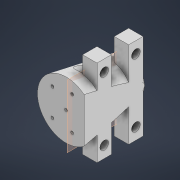
# Autodesk Inventor part: needle module it 5
Saved by Autodesk Inventor 2022 (Build 260153000, 153)
## iProperties
Created: 2023-02-14
Part Number: needle module it 5
Material: Generic
Document SubType Name: Modeling
Designer: Jakob Saugbjerg
Density: 1 g/cm^3
Appearance: Default
Author: Jakob Saugbjerg
Autodesk Inventor part; units mm, degrees
ref_plane "YZ Plane" through (0, 0, 0) normal (1, 0, 0) x (0, 1, 0)
sketch "Sketch1" plane through (0, 0, 0) normal (0, 0, 1) x (1, 0, 0)
  circle A0 centre (0, 0) radius 6.25
  dimension "d1" = 12.5
  constraints: 1 centre point, 1 coincident
  measures "d1" diameter of A0
extrude "Extrusion1" add sketch "Sketch1" along normal blind 21 draft 10
sketch "Sketch2" plane through (0, 0, 0) normal (0, 0, -1) x (-1, 0, 0)
  circle A0 centre (0, 0) radius 6.25 projected
  line L0 (-6.25, 0) -> (-13, 0)
  line L1 (-13, 0) -> (-13, -18)
  line L2 (-13, -18) -> (-6.25, -18)
  line L3 (-6.25, -18) -> (-6.25, 0)
  line L4 (-6.25, 0) -> (-13, 0)
  line L5 (-13, 0) -> (-13, 12)
  line L6 (-13, 12) -> (-6.25, 12)
  line L7 (-6.25, 12) -> (-6.25, 0)
  constraints: 16 end point, 4 parallel, 2 horizontal, 2 perpendicular, 1 horizontal alignment, 1 other
extrude "Extrusion2" cut sketch "Sketch2" against normal blind 21 contours L3 L2 L1 L0 | L0 L5 L6 L7
sketch "Sketch3" plane through (0, 0, 0) normal (0, 0, -1) x (-1, 0, 0)
  circle A0 centre (0, 0) radius 0.5
  dimension "d6" = 1
  constraints: 1 centre point, 1 coincident
  measures "d6" diameter of A0
extrude "Extrusion3" cut sketch "Sketch3" against normal blind 21
sketch "Sketch4" plane through (0, 0, 0) normal (0, 0, -1) x (-1, 0, 0)
  circle A0 centre (0, 0) radius 0.5 projected
  line L0 (0, 0) -> (2.1213, -2.1213)
  line L1 (0, 0) -> (3, 0) construction
  circle A1 centre (2.1213, -2.1213) radius 0.5
  dimension "d9" = 3
  dimension "d10" = 45
  dimension "d11" = 1
  constraints: 4 end point, 1 centre point, 1 coincident, 1 equal length, 1 horizontal
  measures "d9" distance of L0.start L0.end
  measures "d10" angle of L0 L1
  measures "d11" diameter of A1
ref_plane "Work Plane1" through (0, 0, 0) normal (0.7071, -0.7071, 0) x (-0.7071, -0.7071, 0)
sketch "Sketch5" plane through (0, 0, 0) normal (0.7071, -0.7071, 0) x (-0.7071, -0.7071, 0)
  line L0 (3.1664, 0.0352) -> (12.6, 0.0352) construction
  line L1 (9.9529, -21) -> (-9.8965, -21) projected
  line L2 (3.1664, 0.0352) -> (17.0268, 0.0352) construction
  line L3 (3.1664, 0.0352) -> (10.1664, 0.0352) construction
  line L4 (3.0004, 0) -> (10.0004, 0) construction
  line L5 (3.0004, 0) -> (24.3244, 0) construction
  line L6 (3.0004, 0) -> (3.0004, -7) construction
  line L7 (3.0004, -7) -> (3.0004, -7.6423) construction
  line L8 (3.0004, -7.6423) -> (3.0004, -8.3511) construction
  line L9 (-6.25, 0) -> (6.25, 0) projected
  line L10 (3.0004, -8.3511) -> (6.7033, -21) construction
  line L11 (6.7033, -21) -> (6.8441, -21.4575) construction
  spline S0 degree 4 poles (3.0004, 0) (3.0004, -7) (3.0004, -7.6423) (3.0004, -8.3511) (6.7033, -21) (6.8441, -21.4575) knots 1 1 1 1 1 2 3 3 3 3 3
  point P0 (0, 0)
  point P1 (1.0577, -21)
  point P2 (-4.4194, 0)
  constraints: 10 end point, 5 horizontal, 1 perpendicular, 3 other
sketch "Sketch6" plane through (0, 0, 0) normal (0, 0, -1) x (-1, 0, 0)
  line L0 (0, 0) -> (2.1213, 2.1213)
  line L1 (0, 0) -> (3, 0) construction
  circle A0 centre (2.1213, 2.1213) radius 0.5
  dimension "d18" = 3
  dimension "d19" = 45
  dimension "d20" = 1
  constraints: 4 end point, 1 centre point, 1 coincident, 1 equal length, 1 horizontal
  measures "d18" distance of L0.start L0.end
  measures "d19" angle of L1 L0
  measures "d20" diameter of A0
ref_plane "Work Plane2" through (0, 0, 0) normal (-0.7071, -0.7071, 0) x (-0.7071, 0.7071, 0)
sketch "Sketch7" plane through (0, 0, 0) normal (-0.7071, -0.7071, 0) x (-0.7071, 0.7071, 0)
  line L0 (3, 0) -> (24.587, 0) construction
  line L1 (9.9529, -21) -> (-9.8965, -21) projected
  line L2 (3, 0) -> (24.324, 0) construction
  line L3 (-9.8965, -21) -> (1.0577, -21) projected
  line L4 (3, 0) -> (10, 0) construction
  line L5 (3, 0) -> (24.324, 0) construction
  line L6 (3, 0) -> (3, -7) construction
  line L7 (3, -7) -> (3, -7.5001) construction
  line L8 (3, -7.5001) -> (3, -8.6524) construction
  line L9 (3, -8.6524) -> (6.7029, -21) construction
  line L10 (6.7029, -21) -> (7.0715, -22.3013) construction
  spline S0 degree 4 poles (3, 0) (3, -7) (3, -7.5001) (3, -8.6524) (6.7029, -21) (7.0715, -22.3013) knots 1 1 1 1 1 2 3 3 3 3 3
  point P0 (0, 0)
  constraints: 8 end point, 4 horizontal, 1 vertical, 3 other
sketch "Sketch8" plane through (0, 0, 0) normal (0, 0, -1) x (-1, 0, 0)
  line L0 (0, 0) -> (-2.1213, 2.1213)
  line L1 (0, 0) -> (3, 0) construction
  line L2 (-2.1213, 2.1213) -> (-2.1213, -2.8787)
  circle A0 centre (-2.1213, 2.1213) radius 0.5
  dimension "d27" = 3
  dimension "d28" = 135
  dimension "d29" = 5
  dimension "d30" = 45
  dimension "d31" = 1
  constraints: 6 end point, 1 centre point, 1 coincident, 1 equal length, 1 horizontal, 1 vertical
  measures "d27" distance of L0.start L0.end
  measures "d28" angle of L1 L0
  measures "d29" distance of L0.end L2.end
  measures "d30" angle of L2 L0
  measures "d31" diameter of A0
ref_plane "Work Plane3" through (2.1213, 2.1213, 0) normal (1, 0, 0) x (0, -1, 0)
sketch "Sketch15" plane through (6.25, -7.7458, 21) normal (1, 0, 0) x (0, 0, -1)
  line L0 (21, 7.7458) -> (18, 7.7458)
  line L1 (0, -2.2071) -> (0, 17.6986) projected
  line L2 (18, 7.7458) -> (7, 7.7458)
  line L3 (9.5, -7.2542) -> (4.5, -7.2542)
  line L4 (4.5, -7.2542) -> (4.5, 22.7458)
  line L5 (4.5, 22.7458) -> (9.5, 22.7458)
  line L6 (9.5, 22.7458) -> (9.5, -7.2542)
  line L7 (9.5, -7.2542) -> (4.5, 22.7458) construction
  line L8 (4.5, -7.2542) -> (9.5, 22.7458) construction
  line L9 (20.5, -7.2542) -> (15.5, -7.2542)
  line L10 (15.5, -7.2542) -> (15.5, 22.7458)
  line L11 (15.5, 22.7458) -> (20.5, 22.7458)
  line L12 (20.5, 22.7458) -> (20.5, -7.2542)
  line L13 (20.5, -7.2542) -> (15.5, 22.7458) construction
  line L14 (15.5, -7.2542) -> (20.5, 22.7458) construction
  point P0 (0, 0)
  point P1 (0, 15.4916)
  dimension "d46" = 3
  dimension "d47" = 11
  dimension "d48" = 5
  dimension "d49" = 30
  dimension "d50" = 5
  dimension "d51" = 30
  constraints: 28 end point, 4 midpoint, 4 parallel, 3 perpendicular, 2 horizontal, 1 point on line
  measures "d46" distance of L0.start L0.end
  measures "d47" distance of L0.end L2.end
  measures "d48" distance of L4.end L5.end
  measures "d49" distance of L3.end L4.end
  measures "d50" distance of L10.end L11.end
  measures "d51" distance of L9.end L10.end
extrude "Extrusion4" add sketch "Sketch15" against normal blind 5
sketch "Sketch10" plane through (2.1213, 2.1213, 0) normal (1, 0, 0) x (0, -1, 0)
  line L0 (0, 0) -> (15, 0) construction
  line L1 (0, 0) -> (21.324, 0) construction
  line L2 (-4.1287, 0) -> (8.3713, 0) projected
  line L3 (0, 0) -> (7, 0) construction
  line L4 (0, 0) -> (21.324, 0) construction
  line L5 (0, 0) -> (0, -7) construction
  line L6 (0, -7) -> (0, -7.483) construction
  line L7 (0, -7.483) -> (0, -8.2593) construction
  line L8 (0, -8.2593) -> (-3.7029, -21) construction
  line L9 (-3.7029, -21) -> (-3.9552, -21.9025) construction
  spline S0 degree 4 poles (0, 0) (0, -7) (0, -7.483) (0, -8.2593) (-3.7029, -21) (-3.9552, -21.9025) knots 1 1 1 1 1 2 3 3 3 3 3
  point P0 (2.1213, 0)
  point P1 (-5.6245, -21)
  constraints: 8 end point, 4 horizontal, 1 vertical, 3 other
sketch "Sketch11" plane through (0, 0, 0) normal (0, 0, -1) x (-1, 0, 0)
  line L0 (0, 0) -> (-2.1213, -2.1213)
  line L1 (0, 0) -> (3, 0) construction
  circle A0 centre (-2.1213, -2.1213) radius 0.5
  dimension "d38" = 3
  dimension "d39" = 135
  dimension "d40" = 1
  constraints: 4 end point, 1 centre point, 1 coincident, 1 equal length, 1 horizontal
  measures "d38" distance of L0.start L0.end
  measures "d39" angle of L0 L1
  measures "d40" diameter of A0
sketch "Sketch12" plane through (2.1213, 2.1213, 0) normal (1, 0, 0) x (0, -1, 0)
  line L0 (4.2533, 0.2872) -> (19.2533, 0.2872) construction
  line L1 (12.0742, -21) -> (-7.8315, -21) projected
  line L2 (4.2533, 0.2872) -> (25.5773, 0.2872) construction
  line L3 (4.2423, 0) -> (11.2423, 0) construction
  line L4 (4.2423, 0) -> (25.5662, 0) construction
  line L5 (4.2423, 0) -> (4.2423, -7) construction
  line L6 (4.2423, -7) -> (4.2423, -7.5431) construction
  line L7 (4.2423, -7.5431) -> (4.2423, -8.1725) construction
  line L8 (1.6213, 0) -> (2.6213, 0) projected
  line L9 (4.2423, -8.1725) -> (7.9451, -21) construction
  line L10 (7.9451, -21) -> (8.2679, -22.1193) construction
  spline S0 degree 4 poles (4.2423, 0) (4.2423, -7) (4.2423, -7.5431) (4.2423, -8.1725) (7.9451, -21) (8.2679, -22.1193) knots 1 1 1 1 1 2 3 3 3 3 3
  point P0 (2.1213, 0)
  point P1 (9.8671, -21)
  point P2 (-5.6245, -21)
  constraints: 8 end point, 4 horizontal, 1 perpendicular, 3 other
sketch "Sketch16" plane through (6.25, -7.7458, 21) normal (1, 0, 0) x (0, 0, -1)
  line L0 (15.5, -7.2542) -> (20.5, -7.2542) projected
  line L1 (18, -7.2542) -> (18, -3.2542)
  line L2 (18, -7.2542) -> (22, -7.2542) construction
  line L3 (18, -3.2542) -> (18, 18.7458)
  line L4 (18, 18.7458) -> (7, 18.7458)
  line L5 (7, 18.7458) -> (7, -3.2542)
  circle A0 centre (7, -3.2542) radius 1.5
  circle A1 centre (7, 18.7458) radius 1.5
  circle A2 centre (18, -3.2542) radius 1.5
  circle A3 centre (18, 18.7458) radius 1.5
  point P0 (21, 7.7458)
  dimension "d54" = 4
  dimension "d55" = 90
  dimension "d56" = 22
  dimension "d57" = 11
  dimension "d58" = 22
  dimension "d59" = 3
  dimension "d60" = 3
  dimension "d61" = 3
  dimension "d62" = 3
  constraints: 10 end point, 4 centre point, 4 coincident, 3 perpendicular, 1 horizontal, 1 midpoint, 1 point on line, 1 vertical
  measures "d54" distance of L1.start L1.end
  measures "d55" angle of L2 L1
  measures "d56" distance of L1.end L3.end
  measures "d57" distance of L3.end L4.end
  measures "d58" distance of L4.end L5.end
  measures "d59" diameter of A0
  measures "d60" diameter of A1
  measures "d61" diameter of A2
  measures "d62" diameter of A3
extrude "Extrusion5" cut sketch "Sketch16" against normal blind 5
sketch "Sketch17" plane through (1.25, -7.7458, 21) normal (-1, 0, 0) x (0, 0, 1)
  circle A0 centre (-7, -3.2542) radius 1.5 projected
  circle A1 centre (-7, -3.2542) radius 2.95
  circle A2 centre (-7, 18.7458) radius 1.5 projected
  circle A3 centre (-7, 18.7458) radius 2.95
  point P0 (-21, 7.7458)
  dimension "d65" = 5.9
  dimension "d66" = 5.9
  constraints: 2 centre point, 2 coincident
  measures "d65" diameter of A1
  measures "d66" diameter of A3
extrude "Extrusion6" cut sketch "Sketch17" along normal blind 55 contours A0 | A1 | A2 | A3
sweep "Sweep5" cut profiles "Sketch4" path "Sketch5" path curves S0 contours A1
sweep "Sweep6" cut profiles "Sketch6" path "Sketch7" path curves S0
sweep "Sweep7" cut profiles "Sketch8" path "Sketch10" path curves S0
sweep "Sweep8" cut profiles "Sketch11" path "Sketch12" path curves S0
body "Solid1"
